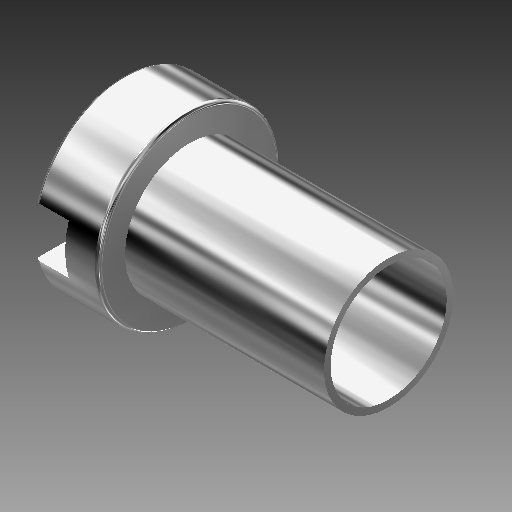
# Autodesk Inventor part: 308-02
Saved by Autodesk Inventor 2019 (Build 230136000, 136)
## iProperties
Company: Autodesk Inc.
Created: 2012-01-27
Part Number: 308-02
Material: Steel
Document SubType Name: Modeling
Designer: Autodesk Inc.
Mass: 0.58937 g
Surface Area: 2.07648 cm^2
Volume: 0.0750789 cm^3
Density: 7.85 g/cm^3
Appearance: Chrome - Polished
Author: Inventor
Autodesk Inventor part; units mm, degrees
ref_plane "YZ Plane" through (0, 0, 0) normal (1, 0, 0) x (0, 1, 0)
sketch "Sketch1" plane through (0, 0, 0) normal (0, 0, 1) x (1, 0, 0)
  line L0 (0, 0) -> (2, 0)
  line L1 (2, 0) -> (2, 2.75)
  line L2 (2, 2.75) -> (0, 2.75)
  line L3 (0, 2.75) -> (0, 0)
  line L4 (2, 0) -> (8, 0)
  line L5 (8, 0) -> (8, 1.95)
  line L6 (8, 1.95) -> (2, 1.95)
  line L7 (2, 1.95) -> (2, 0)
  dimension "d0" = 8
  dimension "d1" = 2
  dimension "d2" = 5.5
  dimension "d3" = 3.9
  constraints: 16 end point, 4 parallel, 2 horizontal, 2 perpendicular
  measures "d0" distance between parallel lines of L5 L3
  measures "d1" distance of L0.start L0.end
  measures "d2" diameter of L2 L0
  measures "d3" diameter of L6 L4
revolve "Revolution1" add sketch "Sketch1" angle 360 about axis through (0, 0, 0) along (1, 0, 0)
ref_plane "Work Plane1" through (1, 0, 0) normal (-1, 0, 0) x (0, 0, 1)
ref_plane "Work Plane2" through (1, 0, 0) normal (1, 0, 0) x (0, 0, -1)
sketch "Sketch2" plane through (0, 0, 0) normal (0, 0, 1) x (1, 0, 0)
  line L0 (0, 0.75) -> (1, 0.75)
  line L1 (1, 0.75) -> (1, -0.75)
  line L2 (1, -0.75) -> (0, -0.75)
  line L3 (0, -0.75) -> (0, 0.75)
  point P0 (0, 0)
  point P1 (0, 0)
  dimension "d7" = 1
  dimension "d8" = 1.5
  constraints: 8 end point, 2 parallel, 1 coincident, 1 horizontal, 1 midpoint, 1 perpendicular
  measures "d7" distance of L1.end L2.end
  measures "d8" distance of L0.end L1.end
extrude "Extrusion1" cut sketch "Sketch2" along normal through all both and the other way through all
hole "Hole1" at (8, 0, 0) direction (-1, 0, 0) diameter 2.013 depth 5 tip angle 118 counterbore diameter 3.5 counterbore depth 3 thread size "M2.5x0.45" class "6H" standard "ANSI Metric M Profile"
fillet "Fillet1" radius 0.12 4 edges at (0, 2.1937, -1.6583) (0, 2.1937, 1.6583) (0, -2.75, 0) (2, -2.75, 0)
body "Solid1"
